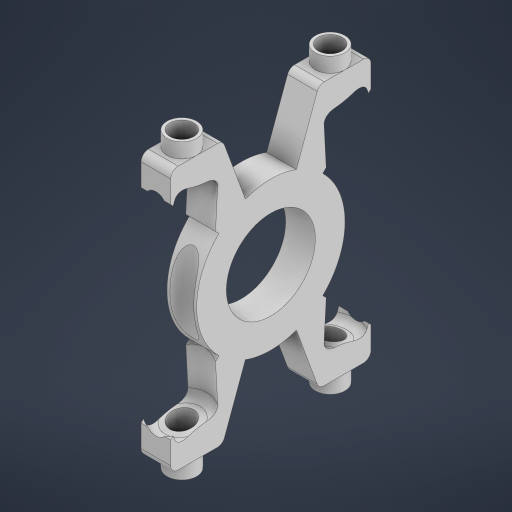
# Autodesk Inventor part: InnerBracket
Saved by Autodesk Inventor 2023 (Build 270158000, 158)
## iProperties
Created: 2023-08-16
Part Number: InnerBracket
Material: Generic
Document SubType Name: Modeling
Designer: Izack Waczko
Density: 1 g/cm^3
Appearance: Default
Author: Izack Waczko
Autodesk Inventor part; units mm, degrees
sketch "Sketch1" plane through (0, 0, 0) normal (1, 0, 0) x (0, 1, 0)
  circle A0 centre (0, 0) radius 6
  circle A1 centre (0, 0) radius 10
  line L0 (-19.75, 10) -> (19.75, 10) construction
  line L1 (19.6718, 0) -> (-19.8282, 0) construction
  line L2 (-19.75, -10) -> (19.75, -10) construction
  line L3 (-19.75, 12) -> (-19.75, 8)
  line L4 (-19.75, -8) -> (-19.75, -12)
  line L5 (19.75, -8) -> (19.75, -12)
  line L6 (19.75, 12) -> (19.75, 8)
  line L7 (17.75, 13.5) -> (17.75, 6.5)
  line L8 (-17.75, 13.5) -> (-17.75, 6.5)
  line L9 (-19.75, 8) -> (-17.75, 8)
  line L10 (-19.75, 12) -> (-17.75, 12)
  line L11 (19.75, 8) -> (17.75, 8)
  line L12 (17.75, 6.5) -> (13.75, 6.5)
  line L13 (13.75, 6.5) -> (13.75, 13.5)
  line L14 (13.75, 13.5) -> (17.75, 13.5)
  line L15 (-17.75, 6.5) -> (-13.75, 6.5)
  line L16 (-13.75, 6.5) -> (-13.75, 13.5)
  line L17 (-13.75, 13.5) -> (-17.75, 13.5)
  line L18 (17.75, -6.5) -> (13.75, -6.5)
  line L19 (13.75, -6.5) -> (13.75, -13.5)
  line L20 (13.75, -13.5) -> (17.75, -13.5)
  line L21 (-13.75, -13.5) -> (-17.75, -13.5)
  line L22 (-13.75, -6.5) -> (-13.75, -13.5)
  line L23 (-17.75, -6.5) -> (-13.75, -6.5)
  line L24 (-17.75, -6.5) -> (-17.75, -13.5)
  line L25 (-19.75, -8) -> (-17.75, -8)
  line L26 (-19.75, -12) -> (-17.75, -12)
  line L27 (17.75, -6.5) -> (17.75, -13.5)
  line L28 (19.75, -8) -> (17.75, -8)
  line L29 (19.75, -12) -> (17.75, -12)
  line L30 (13.75, -6.5) -> (21.4418, -6.5) construction
  line L31 (17.75, -6.5) -> (0, 0)
  line L32 (0, 0) -> (13.75, -13.5)
  line L33 (-17.75, -6.5) -> (0, 0)
  line L34 (0, 0) -> (-17.75, 6.5)
  line L35 (0, 0) -> (17.75, 6.5)
  line L36 (0, 0) -> (13.75, 13.5)
  line L37 (19.75, 12) -> (17.75, 12)
  line L38 (0, 10) -> (0, 0) construction
  line L39 (0, 0) -> (0, -10) construction
  line L40 (0, 0) -> (-13.75, 13.5)
  line L41 (0, 0) -> (-13.75, -13.5)
  point P0 (17.75, 10)
  point P1 (-17.75, 10)
  point P2 (7.1356, -7.0059)
  point P3 (9.3902, -3.4387)
  point P4 (9.3902, 3.4387)
  point P5 (7.1356, 7.0059)
  point P6 (-9.3902, 3.4387)
  point P7 (-9.3902, -3.4387)
  point P8 (-7.1356, -7.0059)
  point P9 (-7.1356, 7.0059)
  dimension "d0" = 12
  dimension "d1" = 20
  dimension "d2" = 39.5
  dimension "d3" = 10
  dimension "d4" = 4
  dimension "d5" = 4
  dimension "d6" = 4
  dimension "d7" = 4
  dimension "d8" = 7
  dimension "d9" = 7
  dimension "d10" = 2
  dimension "d11" = 2
  dimension "d12" = 4
  dimension "d28" = 4
  constraints: 84 end point, 15 point on line, 10 symmetric about line, 8 midpoint, 8 vertical, 7 perpendicular, 5 horizontal, 2 centre point, 2 coincident
  measures "d0" diameter of A0
  measures "d1" diameter of A1
  measures "d2" distance of L0.start L0.end
  measures "d3" distance from line of point (0, 0) L0
  measures "d4" distance of L3.start L3.end
  measures "d5" distance of L4.start L4.end
  measures "d6" distance of L5.start L5.end
  measures "d7" distance of L6.start L6.end
  measures "d8" distance of L7.start L7.end
  measures "d9" distance of L8.start L8.end
  measures "d10" distance between parallel lines of L6 L7
  measures "d11" distance between parallel lines of L3 L8
  measures "d12" distance of L7.end L12.end
  measures "d28" distance of L8.end L16.start
extrude "Extrusion1" add sketch "Sketch1" along normal blind 4 contours A0 L35 A1 L31 | A0 L36 A1 L35 | L31 A1 L32 A0 | A0 L40 A1 L36 | A1 L36 L13 L12 L35 | L32 A1 L41 A0 | L31 L18 L19 L32 A1 | A0 L34 A1 L40 | L33 A1 L34 A0 | A0 L41 A1 L33 | L12 L13 L14 L7 | L27 L20 L19 L18 | A1 L34 L15 L16 L40 | A1 L41 L22 L23 L33 | L7 L37 L6 L11 | L28 L5 L29 L27 | L16 L15 L8 L17 | L23 L22 L21 L24 | L24 L26 L4 L25 | L9 L3 L10 L8
fillet "Fillet1" radius 2 16 edges at (4, 18.75, 8) (4, 18.75, 12) (0, 18.75, 12) (0, 18.75, 8) (4, -18.75, 12) (0, -18.75, 12) (4, -18.75, 8) (0, -18.75, 8) (0, -18.75, -12) (4, -18.75, -12) (0, -18.75, -8) (0, 18.75, -8) (0, 18.75, -12) (4, 18.75, -12) (4, -18.75, -8) (4, 18.75, -8)
sketch "Sketch2" plane through (2, 19.75, 10) normal (0, 1, 0) x (1, 0, 0)
  arc A0 (2, 0) -> (-2, 0) centre (0, 0) ccw projected
  circle A1 centre (0, 0) radius 1.6
  circle A2 centre (0, 20) radius 2 projected
  circle A3 centre (0, 20) radius 1.6
  point P0 (-2, 10)
  dimension "d17" = 3.2
  dimension "d18" = 3.2
  constraints: 2 centre point, 2 coincident
  measures "d17" diameter of A1
  measures "d18" diameter of A3
extrude "Extrusion2" cut sketch "Sketch2" against normal through all contours A1 | A3
ref_plane "Work Plane1" through (2, 0, 0) normal (1, 0, 0) x (0, 0, -1)
sketch "Sketch3" plane through (2, 0, 0) normal (1, 0, 0) x (0, 0, -1)
  line L0 (13.5, -17.75) -> (13.5, -13.75) projected
  line L1 (-13.5, -13.75) -> (13.5, -13.75)
  line L2 (-13.5, 13.75) -> (22.5, 13.75)
  line L3 (-12, 19.75) -> (-8, 19.75) projected
  line L4 (-10, 19.75) -> (-10, 13.75)
  line L5 (8, 19.75) -> (12, 19.75) projected
  line L6 (10, 19.75) -> (10, 13.75)
  line L7 (-8, -19.75) -> (-12, -19.75) projected
  line L8 (-10, -19.75) -> (-10, -13.75)
  line L9 (12, -19.75) -> (8, -19.75) projected
  line L10 (10, -19.75) -> (10, -13.75)
  line L11 (-10, -13.75) -> (-6.5, -13.75)
  line L12 (-6.5, -13.75) -> (-6.5, -4.9653)
  line L13 (-10, -13.75) -> (-13.5, -13.75)
  line L14 (-10, -13.75) -> (-11.1012, -8.4801)
  line L15 (-6.5, -13.75) -> (-7.0059, -7.1356)
  line L16 (-7.0059, -7.1356) -> (-13.5, -13.75) projected
  line L17 (-7.0059, -7.1356) -> (-13.5, -13.75)
  line L18 (-13.5, -13.75) -> (-6.5, -13.75)
  point P0 (0, 0)
  point P1 (-10.6142, -10.8108)
  point P2 (-10.6142, -10.8108)
  dimension "d21" = 3.5
  constraints: 26 end point, 7 point on line, 5 perpendicular, 4 midpoint, 1 collinear, 1 horizontal
  measures "d21" distance of L8.end L11.end
revolve "Revolution1" cut sketch "Sketch3" angle 360 about axis through (2, -13.75, 10) along (0, 0.9788557, 0.2045521) contours L14 L16 L15 L1
fillet "Fillet3" radius 1 3 edges at (2, -15.1516, 13.2071) (3.0506, -13.7838, 6.6616) (0.9494, -13.7838, 6.6616)
ref_plane "Work Plane2" through (0, -17.75, 0) normal (0, 0, 1) x (1, 0, 0)
ref_plane "Work Plane3" through (0, 0, -6.5) normal (0, -1, 0) x (1, 0, 0)
mirror "Mirror1" about plane through (0, -17.75, 0) normal (0, 0, 1) of "Revolution1", "Fillet3"
mirror "Mirror2" about plane through (0, 0, -6.5) normal (0, -1, 0) of "Fillet3", "Revolution1", "Mirror1"
fillet "Fillet6" radius 1 8 edges at (2, 17.75, -6.5) (2, 17.75, -13.5) (2, 17.75, 6.5) (2, 17.75, 13.5) (2, -17.75, 13.5) (2, -17.75, 6.5) (2, -17.75, -6.5) (2, -17.75, -13.5)
body "Solid1"
